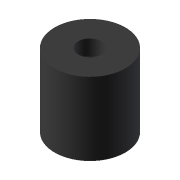
# Autodesk Inventor part: 30_Adapter_M3_nut
Saved by Autodesk Inventor 2019.4 (Build 234330000, 330)
## iProperties
Created: 2020-10-06
Part Number: 30_Adapter_M3_nut
Material: Generic
Document SubType Name: Modeling
Designer: diederichbenedict
Density: 1 g/cm^3
Appearance: Default
Author: diederichbenedict
Autodesk Inventor part; units mm, degrees
ref_plane "YZ Plane" through (0, 0, 0) normal (1, 0, 0) x (0, 1, 0)
ref_plane "XZ Plane" through (0, 0, 0) normal (0, 1, 0) x (-1, 0, 0)
ref_plane "XY Plane" through (0, 0, 0) normal (0, 0, 1) x (1, 0, 0)
sketch "Sketch1" plane through (0, 0, 0) normal (0, 1, 0) x (-1, 0, 0)
  circle A0 centre (0, 0) radius 1.5
  circle A1 centre (0, 0) radius 4.5
  line L0 (-1.6021, 2.775) -> (1.6021, 2.775)
  line L1 (1.6021, 2.775) -> (3.2043, 0)
  line L2 (3.2043, 0) -> (1.6021, -2.775)
  line L3 (1.6021, -2.775) -> (-1.6021, -2.775)
  line L4 (-1.6021, -2.775) -> (-3.2043, 0)
  line L5 (-3.2043, 0) -> (-1.6021, 2.775)
  line L6 (6.3, 0) -> (-6.3, 0) projected
  dimension "d0" = 3
  dimension "d1" = 9
  dimension "d2" = 5.55
  constraints: 12 end point, 3 coincident, 2 centre point, 1 parallel, 13 other
  measures "d0" diameter of A0
  measures "d1" diameter of A1
  measures "d2" distance between parallel lines of L3 L0
extrude "Extrusion1" add sketch "Sketch1" along normal blind 3.3 contours L6 A1 L4 L3 L2 | L1 L0 L5 L6 A1
sketch "Sketch2" plane through (0, 3.3, 0) normal (0, 1, 0) x (1, 0, 0)
  line L0 (-1.6021, -2.775) -> (-3.2043, 0) projected
  line L1 (-3.2043, 0) -> (-1.6021, 2.775) projected
  line L2 (-1.6021, 2.775) -> (1.6021, 2.775) projected
  line L3 (1.6021, 2.775) -> (3.2043, 0) projected
  line L4 (3.2043, 0) -> (1.6021, -2.775) projected
  line L5 (1.6021, -2.775) -> (-1.6021, -2.775) projected
  circle A0 centre (0, 0) radius 4.5 projected
  circle A1 centre (0, 0) radius 1.5
  dimension "d5" = 3
  constraints: 1 centre point, 1 coincident
  measures "d5" diameter of A1
extrude "Extrusion2" add sketch "Sketch2" along normal blind 2 contours L0 L1 L2 L3 L4 L5 | A0
sketch "Sketch3" plane through (0, 0, 0) normal (0, -1, 0) x (1, 0, 0)
  point P0 (0, 0)
sketch "Sketch4" plane through (0, 0, 0) normal (0, -1, 0) x (1, 0, 0)
  line L0 (-3.2043, 0) -> (-1.6021, 2.775) projected
  line L1 (-1.6021, 2.775) -> (1.6021, 2.775) projected
  line L2 (1.6021, 2.775) -> (3.2043, 0) projected
  line L3 (3.2043, 0) -> (1.6021, -2.775) projected
  line L4 (1.6021, -2.775) -> (-1.6021, -2.775) projected
  line L5 (-1.6021, -2.775) -> (-3.2043, 0) projected
  circle A0 centre (0, 0) radius 4.5 projected
  line L6 (3.5218, 0) -> (1.7609, 3.05)
  line L7 (1.7609, 3.05) -> (-1.7609, 3.05)
  line L8 (-1.7609, 3.05) -> (-3.5218, 0)
  line L9 (-3.5218, 0) -> (-1.7609, -3.05)
  line L10 (-1.7609, -3.05) -> (1.7609, -3.05)
  line L11 (1.7609, -3.05) -> (3.5218, 0)
  dimension "d8" = 6.1
  constraints: 12 end point, 5 other
  measures "d8" distance between parallel lines of L9 L6
extrude "Extrusion3" add sketch "Sketch4" along normal blind 4 contours A0
body "Solid1"
